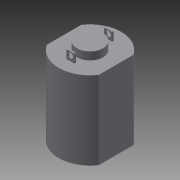
# Autodesk Inventor part: Pololu #2218 Micro Metal Gearmotor HP
Saved by Autodesk Inventor 2014 SP1 (Build 180222100, 222)
## iProperties
Created: 2013-12-20
Part Number: Pololu #2218 Micro Metal Gearmotor HP
Material: Generic
Document SubType Name: Modeling
Designer: JustinIndra
Density: 1 g/cm^3
Appearance: Default
Author: JustinIndra
Autodesk Inventor part; units mm, degrees
ref_plane "YZ Plane" through (0, 0, 0) normal (1, 0, 0) x (0, 1, 0)
ref_plane "XZ Plane" through (0, 0, 0) normal (0, 1, 0) x (-1, 0, 0)
ref_plane "XY Plane" through (0, 0, 0) normal (0, 0, 1) x (1, 0, 0)
sketch "Sketch1" plane through (0, 0, 0) normal (0, 0, 1) x (1, 0, 0)
  circle A0 centre (0, 0) radius 6
  line L0 (-5, 3.3166) -> (-5, -3.3166)
  line L1 (5, 3.3166) -> (5, -3.3166)
  dimension "d0" = 12
  dimension "d1" = 10
  constraints: 4 end point, 4 point on circle, 2 parallel, 1 centre point, 1 coincident, 1 vertical
  measures "d0" diameter of A0
  measures "d1" distance between parallel lines of L1 L0
extrude "Extrusion1" add sketch "Sketch1" along normal blind 15 contours L1 A0 L0
sketch "Sketch2" plane through (0, 0, 15) normal (0, 0, 1) x (1, 0, 0)
  arc A0 (5, 3.3166) -> (-5, 3.3166) centre (0, 0) ccw projected
  circle A1 centre (0, 0) radius 2.5
  dimension "d4" = 5
  constraints: 1 centre point, 1 coincident
  measures "d4" diameter of A1
extrude "Extrusion2" add sketch "Sketch2" along normal blind 1.5
sketch "Sketch3" plane through (0, 0, 15) normal (0, 0, 1) x (1, 0, 0)
  circle A0 centre (0, 0) radius 2.5 projected
  line L0 (-0.775, 3.775) -> (0.775, 3.775)
  line L1 (0.775, 3.775) -> (0.775, 3.475)
  line L2 (0.775, 3.475) -> (-0.775, 3.475)
  line L3 (-0.775, 3.475) -> (-0.775, 3.775)
  point P0 (0, 3.475)
  dimension "d7" = 3.775
  dimension "d8" = 0.3
  dimension "d9" = 1.55
  constraints: 8 end point, 2 parallel, 1 horizontal, 1 midpoint, 1 perpendicular, 1 vertical alignment
  measures "d7" distance from line of A0.centre L0
  measures "d8" distance of L0.end L1.end
  measures "d9" distance of L0.start L0.end
extrude "Extrusion3" add sketch "Sketch3" along normal blind 1.65 contours L0 L1 L2 L3
sketch "Sketch4" plane through (-0.775, 3.775, 15) normal (0, 1, 0) x (1, 0, 0)
  line L0 (1.55, -1.65) -> (0, -1.65) projected
  circle A0 centre (0.775, -0.95) radius 0.5
  point P0 (0.775, 15)
  point P1 (0.775, -1.65)
  dimension "d12" = 1
  dimension "d13" = 0.7
  constraints: 1 centre point, 1 midpoint, 1 vertical alignment
  measures "d12" diameter of A0
  measures "d13" distance from line of L0 A0.centre
extrude "Extrusion4" cut sketch "Sketch4" against normal up to surface (0.3 mm away)
fillet "Fillet1" radius 0.25 2 edges at (0.775, 3.625, 16.65) (-0.775, 3.625, 16.65)
mirror "Mirror1" about plane through (0, 0, 0) normal (0, 1, 0) of "Extrusion3", "Extrusion4", "Fillet1"
body "Solid1"
